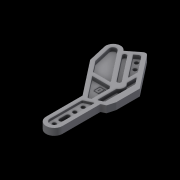
# Autodesk Inventor part: ShinConnector
Saved by Autodesk Inventor 2015 (Build 190159000, 159)
## iProperties
Created: 2014-09-28
Part Number: ShinConnector
Material: Generic
Document SubType Name: Modeling
Designer: Inventor
Mass: 35.771 g
Surface Area: 173.857 cm^2
Volume: 35.771 cm^3
Density: 1 g/cm^3
Appearance: Default
Author: Inventor
Autodesk Inventor part; units mm, degrees
ref_plane "YZ Plane" through (0, 0, 0) normal (1, 0, 0) x (0, 1, 0)
ref_plane "XZ Plane" through (0, 0, 0) normal (0, 1, 0) x (-1, 0, 0)
sketch "Base" plane through (0, 0, 0) normal (0, 0, 1) x (1, 0, 0)
  line L0 (0, -40.5971) -> (0, 168.3327) construction
  arc A0 (-10.75, 0) -> (10.75, 0) centre (0, 0) ccw
  line L1 (10.75, 48) -> (10.75, 0)
  line L2 (-10.75, 0) -> (-10.75, 50)
  line L3 (-19, 62.5716) -> (-16.2211, 52.5512)
  line L4 (-10.75, 50) -> (-16.2211, 52.5512)
  line L5 (-19, 62.5716) -> (-19, 93.5716)
  line L6 (-19, 93.5716) -> (-11.2142, 103.5369)
  line L7 (10.75, 48) -> (46.4584, 93.7046)
  line L8 (46.4584, 93.7046) -> (52.0821, 118.0639)
  arc A1 (52.0821, 118.0639) -> (48.6133, 127.8595) centre (42.6597, 120.2392) ccw
  arc A2 (48.6133, 127.8595) -> (35.0394, 126.1928) centre (42.6597, 120.2392) ccw
  line L9 (34.8364, 125.933) -> (20.2582, 137.3228)
  line L10 (35.0394, 126.1928) -> (34.8364, 125.933)
  arc A3 (20.2582, 137.3228) -> (14.6435, 136.6334) centre (17.7956, 134.1707) ccw
  line L11 (14.6435, 136.6334) -> (-11.2142, 103.5369)
  line L12 (42.6597, 120.2392) -> (48.6133, 127.8595) construction
  dimension "d0" = 142
  dimension "d1" = 155
  dimension "d2" = 21.5
  dimension "d3" = 115
  dimension "d4" = 130.5
  dimension "d7" = 51.5
  dimension "d8" = 18.5
  dimension "d9" = 4
  dimension "d10" = 58
  dimension "d11" = 25
  dimension "d14" = 42
  dimension "d15" = 50
  dimension "d18" = 10
  dimension "d57" = 48
  dimension "d100" = 19
  dimension "d101" = 31
  constraints: 24 end point, 9 point on circle, 7 tangent, 4 centre point, 4 parallel, 3 perpendicular, 1 coincident, 1 collinear, 1 concentric, 1 point on line, 1 vertical
  measures "d0" angle of L7 L1
  measures "d1" angle of L8 L7
  measures "d2" distance between parallel lines of L1 L2
  measures "d3" angle of L4 L2
  measures "d4" angle of L3 L4
  measures "d7" distance between parallel lines of L7 L11
  measures "d8" distance of L9.start L9.end
  measures "d9" radius of A3
  measures "d10" distance of L1.start L7.end
  measures "d11" distance of L7.end L8.end
  measures "d14" distance of L11.start L6.end
  measures "d15" distance of L2.start L2.end
  measures "d18" distance from line of L9 L12.end
  measures "d57" distance of L1.start L1.end
  measures "d100" distance between parallel lines of L5 L0
  measures "d101" distance of L3.start L5.end
extrude "BaseFeature" add sketch "Base" along normal blind 9
ref_plane "SunkenDetailsPlane" through (0, 0, 9) normal (0, 0, 1) x (1, 0, 0)
sketch "SunkenDetails" plane through (0, 0, 9) normal (0, 0, 1) x (1, 0, 0)
  line L0 (0.9151, 89.8249) -> (26.6729, 122.7934)
  line L1 (4.8551, 86.7466) -> (30.613, 119.7151)
  arc A0 (30.613, 119.7151) -> (26.6729, 122.7934) centre (28.6429, 121.2543) ccw
  line L2 (0.9151, 97.9462) -> (24.272, 127.8418)
  line L3 (24.272, 127.8418) -> (20.332, 130.9201)
  line L4 (16.1209, 130.403) -> (0.9151, 110.9404)
  arc A1 (20.332, 130.9201) -> (16.1209, 130.403) centre (18.485, 128.556) ccw
  line L5 (-4, 91.6552) -> (-4, 104.6494)
  line L6 (-4, 104.6494) -> (-11, 95.6898)
  line L7 (-11, 95.6898) -> (-11, 55.6335)
  line L8 (-11, 55.6335) -> (-4, 52.3693)
  line L9 (-4, 77.8836) -> (-4, 52.3693)
  arc A2 (-6.1033, 88.9631) -> (-4, 77.8836) centre (-0.1932, 84.3457) ccw
  line L10 (-6.1033, 88.9631) -> (-4, 91.6552)
  line L11 (5.75, 42.3059) -> (5.75, 0)
  line L12 (-5.75, 47.6685) -> (5.75, 42.3059)
  line L13 (-5.75, 0) -> (-5.75, 47.6685)
  arc A3 (-5.75, 0) -> (5.75, 0) centre (0, 0) ccw
  line L14 (4.6626, 48.3299) -> (26.8264, 76.6983)
  line L15 (3.3496, 76.6983) -> (26.8264, 76.6983)
  line L16 (1, 73.6909) -> (3.3496, 76.6983)
  arc A4 (0.9151, 89.8249) -> (4.8551, 86.7466) centre (2.8851, 88.2857) ccw
  line L17 (7.256, 81.6983) -> (30.7329, 81.6983)
  line L18 (7.256, 81.6983) -> (39.1705, 122.5469)
  line L19 (30.7329, 81.6983) -> (41.8359, 95.9094)
  line L20 (41.8359, 95.9094) -> (47.1112, 118.7594)
  arc A5 (47.1112, 118.7594) -> (39.1705, 122.5469) centre (42.721, 119.7729) ccw
  line L21 (10.75, 0) -> (10.75, 48) construction
  arc A6 (-10.75, 0) -> (10.75, 0) centre (0, 0) ccw construction
  line L22 (10.75, 0) -> (10.75, 48) construction
  line L23 (10.75, 48) -> (46.4584, 93.7046) construction
  line L24 (46.4584, 93.7046) -> (52.0821, 118.0639) construction
  arc A7 (52.0821, 118.0639) -> (35.0394, 126.1928) centre (42.6597, 120.2392) ccw construction
  line L25 (35.0394, 126.1928) -> (34.8364, 125.933) construction
  line L26 (34.8364, 125.933) -> (20.2582, 137.3228) construction
  arc A8 (20.2582, 137.3228) -> (14.6435, 136.6334) centre (17.7956, 134.1707) ccw construction
  line L27 (14.6435, 136.6334) -> (-19, 93.5716) construction
  line L28 (-19, 93.5716) -> (-19, 62.5716) construction
  line L29 (-19, 62.5716) -> (-16.2211, 52.5512) construction
  line L30 (-16.2211, 52.5512) -> (-10.75, 50) construction
  line L31 (-10.75, 50) -> (-10.75, 0) construction
  line L32 (-10.75, 50) -> (-10.75, 0) construction
  line L33 (10.75, 48) -> (46.4584, 93.7046) construction
  line L34 (-19, 93.5716) -> (-19, 62.5716) construction
  line L35 (14.6435, 136.6334) -> (-19, 93.5716) construction
  line L36 (46.4584, 93.7046) -> (52.0821, 118.0639) construction
  line L37 (34.8364, 125.933) -> (20.2582, 137.3228) construction
  arc A9 (-10.75, 0) -> (10.75, 0) centre (0, 0) ccw construction
  line L38 (24.272, 127.8418) -> (30.1821, 123.2243) construction
  line L39 (-10.75, 50) -> (-5.75, 47.6685) construction
  line L40 (-16.2211, 52.5512) -> (-10.75, 50) construction
  line L41 (2.8851, 88.2857) -> (-0.1932, 84.3457) construction
  line L42 (0.9151, 110.9404) -> (0.9151, 97.9462)
  line L43 (0.9151, 97.9462) -> (-4, 91.6552) construction
  line L44 (0.9151, 97.9462) -> (0.9151, 89.8249) construction
  line L45 (39.1705, 122.5469) -> (34.8364, 125.933) construction
  line L46 (1.346, 86.3157) -> (7.256, 81.6983) construction
  line L47 (1, 73.6909) -> (1, 50.0378)
  line L48 (1, 50.0378) -> (4.6626, 48.3299)
  point P0 (-11.2142, 103.5369)
  dimension "d23" = 5
  dimension "d30" = 8
  dimension "d32" = 5
  dimension "d34" = 5
  dimension "d35" = 5
  dimension "d36" = 5
  dimension "d49" = 5
  dimension "d54" = 5
  dimension "d59" = 5
  dimension "d60" = 5
  dimension "d61" = 5
  dimension "d66" = 5
  dimension "d76" = 3
  dimension "d77" = 7
  dimension "d102" = 5
  dimension "d103" = 5
  dimension "d104" = 36
  constraints: 64 end point, 16 parallel, 14 point on circle, 12 collinear, 11 tangent, 6 centre point, 3 vertical, 2 horizontal, 1 concentric, 1 midpoint, 1 perpendicular, 1 point on line
  measures "d23" distance between parallel lines of L31 L13
  measures "d30" distance between parallel lines of L28 L7
  measures "d32" distance between parallel lines of L27 L4
  measures "d34" distance between parallel lines of L2 L0
  measures "d35" distance between parallel lines of L18 L1
  measures "d36" distance between parallel lines of L1 L0
  measures "d49" distance between parallel lines of L17 L15
  measures "d54" distance of L41.start L41.end
  measures "d59" distance between parallel lines of L33 L19
  measures "d60" distance between parallel lines of L24 L20
  measures "d61" distance between parallel lines of L26 L3
  measures "d66" distance of L2.end L3.end
  measures "d76" radius of A1
  measures "d77" distance between parallel lines of L7 L9
  measures "d102" distance between parallel lines of L48 L12
  measures "d103" distance between parallel lines of L47 L9
  measures "d104" distance of L14.start L14.end
extrude "SunkenDetailsFeature" cut sketch "SunkenDetails" against normal blind 5 contours L0 A0 L1 A4 | L42 L4 A1 L3 L2 | L10 A2 L9 L8 L7 L6 L5 | L48 L47 L16 L15 L14 | L18 A5 L20 L19 L17
ref_plane "HolesPlane" through (-11, 95.6898, 6.5) normal (0, 0, 1) x (1, 0, 0)
sketch "Holes" plane through (-11, 95.6898, 6.5) normal (0, 0, 1) x (1, 0, 0)
  circle A0 centre (21.6537, 21.2184) radius 2.5
  circle A1 centre (28.426, 29.8865) radius 2.5
  circle A2 centre (11, -57.6898) radius 2.5
  circle A3 centre (11, -68.6898) radius 2.5
  line L0 (8.5, -77.6898) -> (8.5, -86.6898)
  arc A4 (8.5, -86.6898) -> (13.5, -86.6898) centre (11, -86.6898) ccw
  line L1 (13.5, -86.6898) -> (13.5, -77.6898)
  arc A5 (13.5, -77.6898) -> (8.5, -77.6898) centre (11, -77.6898) ccw
  circle A6 centre (11, -95.6898) radius 2.5
  line L2 (11.9151, 15.2506) -> (27.1209, 34.7132) construction
  line L3 (35.272, 32.152) -> (11.9151, 2.2564) construction
  line L4 (21.6537, 21.2184) -> (28.426, 29.8865) construction
  line L5 (31.332, 35.2303) -> (35.272, 32.152) projected
  arc A7 (0.25, -95.6898) -> (21.75, -95.6898) centre (11, -95.6898) ccw construction
  line L6 (0.25, -45.6898) -> (0.25, -95.6898) construction
  line L7 (21.75, -95.6898) -> (21.75, -47.6898) construction
  line L8 (11, -57.6898) -> (11, -95.6898) construction
  dimension "d83" = 5
  dimension "d84" = 9
  dimension "d85" = 9
  dimension "d86" = 9
  dimension "d87" = 11
  dimension "d88" = 8
  dimension "d89" = 11
  dimension "d90" = 4
  dimension "d91" = 6
  constraints: 8 end point, 7 centre point, 6 equal radius, 4 point on circle, 3 point on line, 3 tangent, 2 parallel, 1 concentric, 1 vertical
  measures "d83" diameter of A2
  measures "d84" distance of L0.start L0.end
  measures "d85" distance of A6.centre A4.centre
  measures "d86" distance of A3.centre A5.centre
  measures "d87" distance of L8.start A3.centre
  measures "d88" distance between parallel lines of L2 L3
  measures "d89" distance of L4.start L4.end
  measures "d90" distance between parallel lines of L2 L4
  measures "d91" distance from line of L4.end L5
extrude "HolesFeature" cut sketch "Holes" against normal through all
extrude "SunkenDetailFeature" cut sketch "SunkenDetails" against normal blind 3 contours L11 A3 L13 L12
chamfer "DetailChamfersFeature" distance 1 angle 45 9 edges at (0.9151, 97.9462, 6.5) (-4, 104.6494, 6.5) (-11, 95.6898, 6.5) (-5.75, 47.6685, 7.5) (5.75, 42.3059, 7.5) (-4, 52.3693, 6.5) (7.256, 81.6983, 6.5) (4.6626, 48.3299, 6.5) (-11, 55.6335, 6.5)
sketch "Logo" plane through (0, 0, 4) normal (0, 0, 1) x (1, 0, 0)
  line L0 (3.3496, 76.6983) -> (26.8264, 76.6983) construction
  line L1 (1, 50.0378) -> (1, 73.6909) construction
  line L2 (8, 73.6983) -> (8, 66.1983)
  line L3 (10, 68.1983) -> (10, 71.6983)
  line L4 (13.5, 65.1983) -> (3, 65.1983)
  line L5 (3, 74.6983) -> (14.5, 74.6983)
  line L6 (10, 71.6983) -> (11.5, 71.6983)
  line L7 (11.5, 71.6983) -> (11.5, 68.1983)
  line L8 (13.5, 73.6983) -> (8, 73.6983)
  line L9 (13.5, 66.1983) -> (13.5, 73.6983)
  line L10 (11.5, 68.1983) -> (10, 68.1983)
  line L11 (8, 66.1983) -> (13.5, 66.1983)
  line L12 (13.5, 66.1983) -> (13.5, 65.1983)
  line L13 (13.5, 66.1983) -> (14.5, 66.1983)
  line L14 (3, 65.1983) -> (3, 74.6983)
  line L15 (6, 66.1983) -> (4, 66.1983)
  line L16 (4, 73.6983) -> (6, 73.6983)
  line L17 (4, 66.1983) -> (4, 73.6983)
  line L18 (6, 73.6983) -> (6, 66.1983)
  line L19 (14.5, 74.6983) -> (14.5, 66.1983)
  dimension "d126" = 1
  dimension "d127" = 1
  dimension "d128" = 1
  dimension "d129" = 1
  dimension "d130" = 2
  dimension "d131" = 1.5
  dimension "d132" = 2
  dimension "d133" = 2
  dimension "d134" = 2
  dimension "d135" = 2
  dimension "d136" = 2
  dimension "d137" = 2
  dimension "d138" = 2
  dimension "d139" = 3.5
  constraints: 36 end point, 13 perpendicular, 2 collinear, 1 parallel
  measures "d126" distance between parallel lines of L5 L16
  measures "d127" distance between parallel lines of L14 L17
  measures "d128" distance between parallel lines of L19 L9
  measures "d129" distance between parallel lines of L4 L11
  measures "d130" distance between parallel lines of L2 L18
  measures "d131" distance between parallel lines of L7 L3
  measures "d132" distance between parallel lines of L2 L3
  measures "d133" distance between parallel lines of L9 L7
  measures "d134" distance between parallel lines of L17 L18
  measures "d135" distance between parallel lines of L0 L5
  measures "d136" distance between parallel lines of L1 L14
  measures "d137" distance between parallel lines of L8 L6
  measures "d138" distance between parallel lines of L11 L10
  measures "d139" distance of L7.start L7.end
extrude "LogoFeature" cut sketch "Logo" against normal blind 1
mirror "LeftMirror" about plane through (0, 0, 0) normal (1, 0, 0) remove original yes
